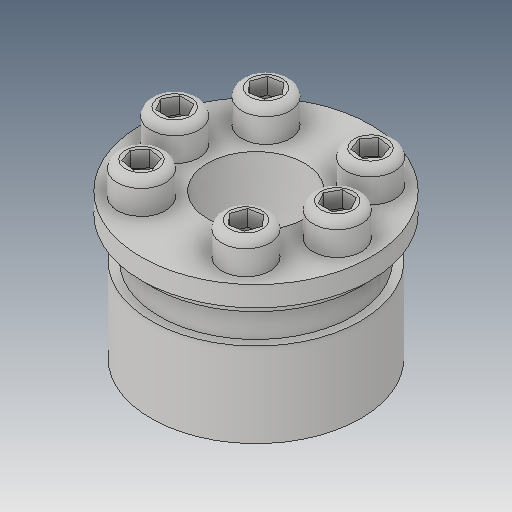
# Autodesk Inventor part: メカロック
Saved by Autodesk Inventor 2020.3 (Build 243373000, 373)
## iProperties
Part Number: メカロック
Material: 一般
Document SubType Name: Modeling
Designer: highs
Density: 1 g/cm^3
Appearance: 既定
Stock Number: 要調査
Author: highs
Autodesk Inventor part; units mm, degrees
ref_plane "YZ Plane" through (0, 0, 0) normal (1, 0, 0) x (0, 1, 0)
ref_plane "XZ Plane" through (0, 0, 0) normal (0, 1, 0) x (-1, 0, 0)
ref_plane "XY Plane" through (0, 0, 0) normal (0, 0, 1) x (1, 0, 0)
sketch "スケッチ1" plane through (0, 0, 0) normal (0, 0, 1) x (1, 0, 0)
  line L0 (0, 0) -> (0, 18)
  line L1 (0, 18) -> (14.25, 18)
  line L2 (14.25, 18) -> (14.25, 15.5)
  line L3 (14.25, 15.5) -> (13, 15.5)
  line L4 (13, 15.5) -> (13, 14.2)
  line L5 (13, 14.2) -> (12, 14.2)
  line L6 (12, 14.2) -> (12, 10.5)
  line L7 (12, 10.5) -> (13, 10.5)
  line L8 (13, 10.5) -> (13, 0)
  line L9 (13, 0) -> (0, 0)
  dimension "d0" = 10.5
  dimension "d1" = 15.5
  dimension "d2" = 18
  dimension "d3" = 14.25
  dimension "d4" = 13
  dimension "d5" = 1.3
  dimension "d6" = 1
  constraints: 20 end point, 6 perpendicular, 2 point on line, 2 vertical, 1 horizontal
  measures "d0" distance of L7.end L8.end
  measures "d1" distance between parallel lines of L9 L3
  measures "d2" distance between parallel lines of L9 L1
  measures "d3" distance of L0.end L1.end
  measures "d4" distance between parallel lines of L0 L8
  measures "d5" distance of L3.end L4.end
  measures "d6" distance of L4.end L5.end
revolve "回転1" add sketch "スケッチ1" angle 360 about axis through (0, 0, 0) along (0, 1, 0)
sketch "スケッチ2" plane through (0, 18, 0) normal (0, 1, 0) x (1, 0, 0)
  circle A0 centre (0, 0) radius 10.1 construction
  circle A1 centre (0, 0) radius 6
  dimension "d8" = 12
  dimension "d9" = 20.2
  constraints: 2 centre point, 2 coincident
  measures "d8" diameter of A1
  measures "d9" diameter of A0
extrude "押し出し1" cut sketch "スケッチ2" against normal through all
sketch "スケッチ3" plane through (0, 18, 0) normal (0, 1, 0) x (1, 0, 0)
  circle A0 centre (0, 0) radius 10.1 construction
  line L0 (0, 0) -> (0, 14.25) construction
  circle A1 centre (0, 0) radius 14.25 construction
  circle A2 centre (-10.1, 0) radius 3
  line L1 (0, 0) -> (-14.25, 0) construction
  dimension "d13" = 20.2
  dimension "d12" = 6
  constraints: 4 end point, 2 point on circle, 1 centre point, 1 coincident, 1 horizontal, 1 horizontal alignment, 1 point on line, 1 vertical, 2 other
  measures "d12" diameter of A2
extrude "押し出し2" add sketch "スケッチ3" along normal blind 4
fillet "フィレット1" radius 1 1 edges at (-13.1, 22, 0)
sketch "スケッチ4" plane through (-10.1, 22, 0) normal (0, 1, 0) x (1, 0, 0)
  circle A0 centre (0, 0) radius 2 projected
  line L0 (-0.866, 1.5) -> (0.866, 1.5)
  line L1 (0.866, 1.5) -> (1.7321, 0)
  line L2 (1.7321, 0) -> (0.866, -1.5)
  line L3 (0.866, -1.5) -> (-0.866, -1.5)
  line L4 (-0.866, -1.5) -> (-1.7321, 0)
  line L5 (-1.7321, 0) -> (-0.866, 1.5)
  point P0 (10.1, 0)
  dimension "d21" = 3
  constraints: 12 end point, 1 coincident, 1 horizontal, 13 other
  measures "d21" distance between parallel lines of L4 L1
extrude "押し出し3" cut sketch "スケッチ4" against normal blind 2 contours L0 L1 L2 L3 L4 L5
pattern_circular "円形状パターン1" count 3 over 100 about axis through (0, 18, 0) along (0, -1, 0) of "押し出し3", "フィレット1", "押し出し2" both ways yes
pattern_circular "円形状パターン2" count 2 over 360 about axis through (0, 18, 0) along (0, -1, 0) of "押し出し2", "フィレット1", "押し出し3", "円形状パターン1"
